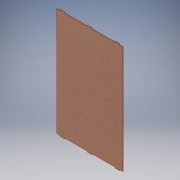
# Autodesk Inventor part: Superior_3mm
Saved by Autodesk Inventor 2017 (Build 210142000, 142)
## iProperties
Created: 2017-10-02
Part Number: Superior_3mm
Material: Wood (Oak)
Document SubType Name: Modeling
Designer: Felipe
Density: 0.76 g/cm^3
Appearance: White Oak - Natural Medium Gloss
Author: Felipe
Autodesk Inventor part; units mm, degrees
ref_plane "YZ Plane" through (0, 0, 0) normal (1, 0, 0) x (0, 1, 0)
ref_plane "XZ Plane" through (0, 0, 0) normal (0, 1, 0) x (-1, 0, 0)
ref_plane "XY Plane" through (0, 0, 0) normal (0, 0, 1) x (1, 0, 0)
sketch "Sketch1" plane through (0, 0, 0) normal (0, 1, 0) x (-1, 0, 0)
  line L0 (0, 0) -> (550, 0) construction
  line L1 (550, 0) -> (550, -900)
  line L2 (550, -900) -> (0, -900) construction
  line L3 (0, -900) -> (0, 0)
  line L4 (520, 0) -> (485, 0) construction
  line L5 (485, 0) -> (485, 7.3489)
  line L6 (485, 7.3489) -> (520, 7.3489)
  line L7 (520, 7.3489) -> (520, 0)
  line L8 (293, 0) -> (258, 0) construction
  line L9 (258, 0) -> (258, 7.3489)
  line L10 (258, 7.3489) -> (293, 7.3489)
  line L11 (293, 7.3489) -> (293, 0)
  line L12 (550, 0) -> (520, 0)
  line L13 (0, 0) -> (258, 0) construction
  line L14 (485, 0) -> (293, 0)
  line L15 (0, -450) -> (550, -450) construction
  line L16 (485, -900) -> (485, -907.3489)
  line L17 (485, -907.3489) -> (520, -907.3489)
  line L18 (520, -907.3489) -> (520, -900)
  line L19 (258, -900) -> (258, -907.3489)
  line L20 (258, -907.3489) -> (293, -907.3489)
  line L21 (293, -907.3489) -> (293, -900)
  line L22 (0, -900) -> (258, -900) construction
  line L23 (293, -900) -> (485, -900)
  line L24 (520, -900) -> (550, -900)
  line L25 (65, 0) -> (30, 0) construction
  line L26 (30, 0) -> (30, 7.3489)
  line L27 (30, 7.3489) -> (65, 7.3489)
  line L28 (65, 7.3489) -> (65, 0)
  line L29 (258, 0) -> (65, 0)
  line L30 (30, 0) -> (0, 0)
  line L31 (65, -900) -> (30, -900) construction
  line L32 (30, -900) -> (30, -907.3489)
  line L33 (30, -907.3489) -> (65, -907.3489)
  line L34 (65, -907.3489) -> (65, -900)
  line L35 (258, -900) -> (65, -900)
  line L36 (30, -900) -> (0, -900)
  dimension "d0" = 900
  dimension "d1" = 550
  dimension "d4" = 35
  dimension "d5" = 35
  dimension "d6" = 192
  dimension "d7" = 30
  dimension "d8" = 258
  dimension "d9" = 193
  constraints: 74 end point, 12 symmetric about line, 8 collinear, 8 parallel, 6 perpendicular, 5 point on line, 4 horizontal, 2 equal length, 2 midpoint
  measures "d0" distance of L0.end L1.end
  measures "d1" distance of L0.start L0.end
  measures "d4" distance of L5.end L6.end
  measures "d5" distance of L9.end L10.end
  measures "d6" distance between parallel lines of L5 L11
  measures "d7" distance between parallel lines of L1 L7
  measures "d8" distance between parallel lines of L3 L9
  measures "d9" distance between parallel lines of L28 L9
extrude "Extrusion1" add sketch "Sketch1" along normal blind 3
body "Solid1"
